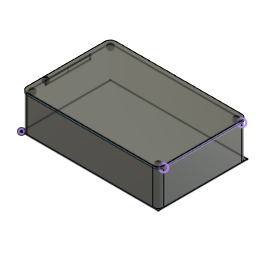
Fusion360 Norm Box Template (Autodesk Fusion 360 design; units mm, degrees)
Autodesk Fusion 360 part; units mm, degrees
sketch "Base" plane through (0, 0, 0) normal (0, 1, 0) x (1, 0, 0) in component "Case"
  line L0 (0, 0) -> (100, 0)
  line L1 (100, 0) -> (100, 65)
  line L2 (100, 65) -> (0, 65)
  line L3 (0, 65) -> (0, 0)
  dimension "d6" = 100
  dimension "d7" = 65
  constraint horizontal L0
  constraint vertical L1
  constraint horizontal L2
  constraint vertical L3
  constraint coincident L0.start L3.end
  measures "d6" distance of L0.start L0.end
  measures "d7" distance of L0.start L2.end
extrude "Extrude1" add sketch "Base" along normal blind 25 makes body 1 in component "Case"
fillet "Fillet1" radius 4 4 edges at (100, 12.5, 0) (0, 12.5, 0) (100, 12.5, -65) (0, 12.5, -65) on bodies 1 in component "Case"
shell "Shell1" thickness 1.5 removed faces 1 at (65.3333, 25, -21.6667) on bodies 1 in component "Case"
sketch "Knob" plane through (1.5, 0, 0) normal (1, 0, 0) x (0, 0, -1) in component "Case"
  line L0 (61, 1.5) -> (61, 25)
  line L1 (61, 25) -> (4, 25)
  line L2 (4, 25) -> (4, 1.5)
  line L3 (4, 1.5) -> (61, 1.5)
  line L4 (16.25, 25) -> (48.75, 25)
  line L5 (48.75, 25) -> (48.75, 22)
  line L6 (48.75, 22) -> (16.25, 22)
  line L7 (16.25, 22) -> (16.25, 25)
  line L8 (32.5, 25) -> (32.5, 22) construction
  dimension "d12" = 32.5
  dimension "d13" = 3
  constraint horizontal L4
  constraint vertical L5
  constraint horizontal L6
  constraint vertical L7
  constraint coincident L1 L4.start
  constraint midpoint L1 L8.start
  constraint midpoint L6 L8.end
  constraint vertical L8
  measures "d12" distance of L5.end L6.end
  measures "d13" distance of L4.end L5.end
extrude "Extrude2" add sketch "Knob" along normal blind 6 draft -45 contours L1 L4 L5 L6 L7 bodies 1 in component "Case"
ref_plane "WorkPlane2" through (50, 12.5, -32.5) normal (-1, 0, 0) x (0, 0, 1) in component "Case"
mirror "Mirror1" about plane through (50, 12.5, -32.5) normal (-1, 0, 0) of "Extrude2" in component "Case"
sketch "Top" plane through (0, 25, 0) normal (0, 1, 0) x (-1, 0, 0) in component "Top Cover"
  line L0 (-100, -4) -> (-100, -61)
  arc A0 (-100, -61) -> (-96, -65) centre (-96, -61) ccw
  line L1 (-96, -65) -> (-4, -65)
  arc A1 (-4, -65) -> (0, -61) centre (-4, -61) ccw
  line L2 (0, -61) -> (0, -4)
  arc A2 (0, -4) -> (-4, 0) centre (-4, -4) ccw
  line L3 (-4, 0) -> (-96, 0)
  arc A3 (-96, 0) -> (-100, -4) centre (-96, -4) ccw
  line L4 (-98.5, -16.25) -> (-98.5, -4)
  arc A4 (-96, -1.5) -> (-98.5, -4) centre (-96, -4) ccw
  line L5 (-96, -1.5) -> (-4, -1.5)
  arc A5 (-1.5, -4) -> (-4, -1.5) centre (-4, -4) ccw
  line L6 (-1.5, -4) -> (-1.5, -16.25)
  line L7 (-1.5, -16.25) -> (-1.5, -48.75)
  line L8 (-1.5, -48.75) -> (-1.5, -61)
  arc A6 (-4, -63.5) -> (-1.5, -61) centre (-4, -61) ccw
  line L9 (-4, -63.5) -> (-96, -63.5)
  arc A7 (-98.5, -61) -> (-96, -63.5) centre (-96, -61) ccw
  line L10 (-98.5, -61) -> (-98.5, -48.75)
  line L11 (-98.5, -48.75) -> (-98.5, -16.25)
extrude "Extrude1'" add sketch "Top" along normal blind 1.5 separate body contours L0 A0 L1 A1 L2 A2 L3 A3 | L4 A4 L5 A5 L6 L7 L8 A6 L9 A7 L10 L11 makes body 2 in component "Top Cover"
sketch "Lip" plane through (0, 25, 0) normal (0, -1, 0) x (1, 0, 0) in component "Top Cover"
  arc A0 (100, -4) -> (96, 0) centre (96, -4) ccw
  line L0 (96, 0) -> (4, 0)
  arc A1 (4, 0) -> (0, -4) centre (4, -4) ccw
  line L1 (0, -4) -> (0, -61)
  arc A2 (0, -61) -> (4, -65) centre (4, -61) ccw
  line L2 (4, -65) -> (96, -65)
  arc A3 (96, -65) -> (100, -61) centre (96, -61) ccw
  line L3 (100, -61) -> (100, -4)
  line L4 (98.3, -61) -> (98.3, -4)
  arc A4 (98.3, -4) -> (96, -1.7) centre (96, -4) ccw
  line L5 (96, -1.7) -> (4, -1.7)
  arc A5 (4, -1.7) -> (1.7, -4) centre (4, -4) ccw
  line L6 (1.7, -4) -> (1.7, -61)
  arc A6 (1.7, -61) -> (4, -63.3) centre (4, -61) ccw
  line L7 (4, -63.3) -> (96, -63.3)
  arc A7 (96, -63.3) -> (98.3, -61) centre (96, -61) ccw
  line L8 (100, -4) -> (100, -61)
  dimension "d19" = 1.7
  dimension "d31" = 1.7
  measures "d31" distance of L4 L8
extrude "Extrude2'" add sketch "Lip" along normal blind 3 contours L4 A4 L5 A5 L6 A6 L7 A7 bodies 2 in component "Top Cover"
extrude "Extrude3" cut sketch "Knob" along normal blind 3 draft -45 from surface at 0.2 contours L1 L4 L5 L6 L7 bodies 2 in component "Top Cover"
ref_plane "WorkPlane2" through (50, 0, 0) normal (1, 0, 0) x (0, 1, 0) in component "Top Cover"
mirror "Mirror1'" about plane through (50, 0, 0) normal (1, 0, 0) of "Extrude3" in component "Top Cover"
shell "Shell1'" thickness 1.5 removed faces 1 at (66.1, 22, -27.0833) on bodies 2 in component "Top Cover"
chamfer "Chamfer1" distance 0.6 angle 45 2 edges at (1.7, 22, -32.5) (98.3, 22, -32.5) on bodies 2 in component "Top Cover"
component "Enclosure" placed x (1, 0, 0) y (0, 1, 0) z (0, 0, 1) at (0, 0, 0)
component "Case" placed x (1, 0, 0) y (0, 1, 0) z (0, 0, 1) at (0, 0, 0) in component "Enclosure"
component "Top Cover" placed x (1, 0, 0) y (0, 1, 0) z (0, 0, 1) at (0, 0, 0) in component "Enclosure"
equation "Width = 65 mm"
equation "length = 100 mm"
equation "heigth = 25 mm"
equation "shell = 1.5 mm"
equation "gap = 0.2 mm"
equation "d6 = length"
equation "d7 = Width"
equation "d8 = heigth"
equation "d11 = shell"
equation "d12 = Width / 2"
equation "d13 = shell * 2"
equation "d17 = shell"
equation "d19 = shell + gap"
equation "d20 = shell * 2"
equation "d23 = shell * 2"
equation "d26 = shell"
equation "d33 = length / 2"
